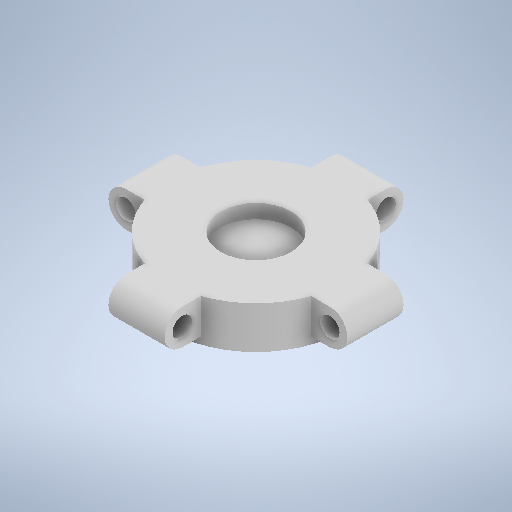
# Autodesk Inventor part: scrambler_vertical_cap
Saved by Autodesk Inventor 2025.2 (Build 292293000, 293)
## iProperties
Created: 2025-10-14
Part Number: scrambler_vertical_cap
Material: Generic
Document SubType Name: Modeling
Designer: pascu
Density: 1 g/cm^3
Appearance: Default
Author: pascu
Autodesk Inventor part; units mm, degrees
ref_plane "YZ Plane" through (0, 0, 0) normal (1, 0, 0) x (0, 1, 0)
ref_plane "XZ Plane" through (0, 0, 0) normal (0, 1, 0) x (-1, 0, 0)
ref_plane "XY Plane" through (0, 0, 0) normal (0, 0, 1) x (1, 0, 0)
sketch "Sketch1" plane through (0, 0, 0) normal (0, 1, 0) x (-1, 0, 0)
  circle A0 centre (0, 0) radius 7.9375
  dimension "d0" = 15.875
  constraints: 1 centre point, 1 coincident
  measures "d0" diameter of A0
extrude "Extrusion1" add sketch "Sketch1" along normal blind 3.81
sketch "Sketch2" plane through (0, 3.81, 0) normal (0, 1, 0) x (1, 0, 0)
  circle A0 centre (0, 0) radius 3.175
  dimension "d3" = 6.35
  constraints: 1 centre point, 1 coincident
  measures "d3" diameter of A0
sketch "Sketch3" plane through (0, 0, 0) normal (1, 0, 0) x (0, 1, 0)
  line L0 (0.635, -2.54) -> (3.81, -2.54)
  line L1 (3.81, -2.54) -> (3.81, 2.54)
  line L2 (3.81, 2.54) -> (0.635, 2.54)
  line L3 (3.81, -7.9375) -> (3.81, 7.9375) projected
  line L4 (0.635, 2.54) -> (0.635, -2.54)
  point P0 (0, 0)
  dimension "d9" = 3.175
  dimension "d20" = 3.175
  constraints: 8 end point, 1 collinear, 1 perpendicular, 1 vertical
  measures "d9" distance of L0.start L0.end
  measures "d20" distance of L1.end L2.end
extrude "Extrusion3" add sketch "Sketch3" along normal mid plane 21.59
fillet "Fillet1" radius 1.5875 4 edges at (10.795, 3.81, 0) (-10.795, 3.81, 0) (10.795, 0.635, 0) (-10.795, 0.635, 0)
sketch "Sketch6" plane through (-7.5201, 0.635, 2.54) normal (0, 0, 1) x (1, 0, 0)
  arc A0 (-1.6874, 3.175) -> (-1.6874, 0) centre (-1.6874, 1.5875) ccw projected
  circle A1 centre (-1.6874, 1.5875) radius 0.889
  arc A2 (16.7276, 0) -> (16.7276, 3.175) centre (16.7276, 1.5875) ccw projected
  circle A3 centre (16.7276, 1.5875) radius 0.889
  point P0 (7.5201, -0.635)
  dimension "d25" = 1.778
  dimension "d26" = 1.778
  constraints: 2 centre point, 2 coincident
  measures "d25" diameter of A1
  measures "d26" diameter of A3
extrude "Extrusion7" cut sketch "Sketch6" against normal through all
pattern_circular "Circular Pattern3" count 2 over 90 about axis through (0, 0, 0) along (0, 1, 0) of "Extrusion3", "Fillet1", "Extrusion7"
extrude "Extrusion8" cut sketch "Sketch2" against normal blind 1.27
body "Solid1"
